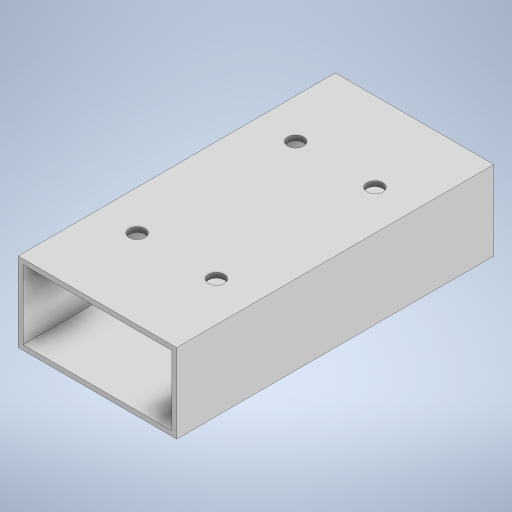
# Autodesk Inventor part: CrossBar
Saved by Autodesk Inventor 2023 (Build 270158000, 158)
## iProperties
Created: 2023-01-22
Part Number: CrossBar
Material: Generic
Document SubType Name: Modeling
Designer: matth
Density: 1 g/cm^3
Appearance: Default
Author: matth
Autodesk Inventor part; units mm, degrees
ref_plane "YZ Plane" through (0, 0, 0) normal (1, 0, 0) x (0, 1, 0)
ref_plane "XZ Plane" through (0, 0, 0) normal (0, 1, 0) x (-1, 0, 0)
ref_plane "XY Plane" through (0, 0, 0) normal (0, 0, 1) x (1, 0, 0)
sketch "Sketch1" plane through (0, 0, 0) normal (0, 0, 1) x (1, 0, 0)
  line L0 (0, 0) -> (50.8, 0)
  line L1 (50.8, 0) -> (50.8, 25.4)
  line L2 (50.8, 25.4) -> (0, 25.4)
  line L3 (0, 25.4) -> (0, 0)
  dimension "d0" = 50.8
  dimension "d1" = 25.4
  constraints: 8 end point, 2 parallel, 1 horizontal, 1 perpendicular
  measures "d0" distance of L2.end L1.end
  measures "d1" distance of L1.end L0.end
extrude "Extrusion1" add sketch "Sketch1" along normal blind 101.6
shell "Shell1" thickness 1.5875 removed faces 2 at (16.9333, 8.4667, 0) at (16.9333, 8.4667, 101.6)
sketch "Sketch2" plane through (0, 25.4, 0) normal (0, 1, 0) x (1, 0, 0)
  line L0 (0, 0) -> (50.8, 0)
  line L1 (50.8, 0) -> (50.8, -101.6)
  line L2 (50.8, -101.6) -> (0, -101.6)
  line L3 (0, -101.6) -> (0, 0)
  circle A0 centre (12.7, -25.4) radius 2.5797
  circle A1 centre (38.1, -25.4) radius 2.5797
  circle A2 centre (12.7, -76.2) radius 2.5797
  circle A3 centre (38.1, -76.2) radius 2.5797
  dimension "d5" = 50.8
  dimension "d6" = 101.6
  dimension "d9" = 25.4
  dimension "d12" = 50.8
  dimension "d15" = 12.7
  dimension "d16" = 25.4
  dimension "d17" = 5.1594
  constraints: 8 end point, 4 centre point, 2 horizontal, 2 parallel, 1 perpendicular, 1 vertical, 6 other
  measures "d5" distance of L1.end L2.end
  measures "d6" distance of L0.end L1.end
  measures "d9" distance of A0.centre A1.centre
  measures "d12" distance of A0.centre A2.centre
  measures "d15" distance from line of L3 A0.centre
  measures "d16" distance from line of A0.centre L0
  measures "d17" diameter of A0
extrude "Extrusion2" cut sketch "Sketch2" against normal through all contours A0 | A1 | A2 | A3
equation "\"d2\" = Length"
equation "\"Length\" = 101.6"
body "Solid1"
